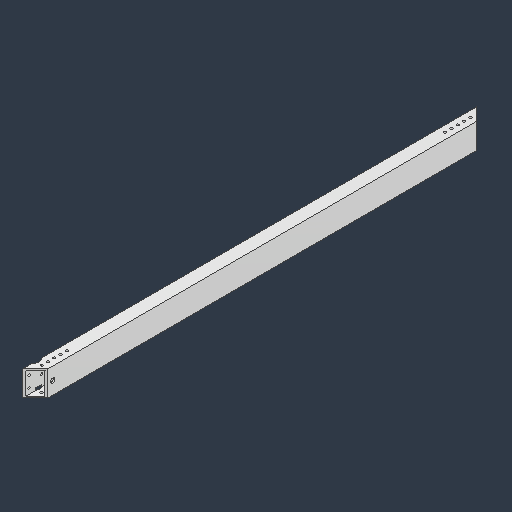
# Autodesk Inventor part: TUBE,ELEVATOR,SIDE,STAGE1
Saved by Autodesk Inventor 2024.3 (Build 283343000, 343)
## iProperties
Created: 2025-01-27
Part Number: TUBE,ELEVATOR,SIDE,STAGE1
Material: Aluminum 6061 T6 0 Cold Formed
Document SubType Name: Modeling
Designer: Jthib
Density: 2.7 g/cm^3
Appearance: Satin
Mass: 1058.01 g
Surface Area: 2496.4 cm^2
Volume: 391.854 cm^3
Mfg Approved By: John.Thibert
ILogicPurgeVersion: 0.0.0.0
OnSaveVersion: 3.4.3.0
OnSaveAssembly: COREAutomationManager
ModelCat: Uncategorized
MaterialName: Aluminum 6061 T6 0 Cold Formed
CN_MASS: 1.06
Author: Jthib
Autodesk Inventor part; units mm, degrees
ref_plane "YZ Plane" through (0, 0, 0) normal (1, 0, 0) x (0, 1, 0)
ref_plane "XZ Plane" through (0, 0, 0) normal (0, 1, 0) x (-1, 0, 0)
ref_plane "XY Plane" through (0, 0, 0) normal (0, 0, 1) x (1, 0, 0)
sketch "Sketch1" plane through (0, 0, 0) normal (0, 0, 1) x (1, 0, 0)
  line L0 (-12.7, -25.4) -> (12.7, -25.4)
  line L1 (12.7, -25.4) -> (12.7, 25.4)
  line L2 (12.7, 25.4) -> (-12.7, 25.4)
  line L3 (-12.7, 25.4) -> (-12.7, -25.4)
  line L4 (-12.7, -25.4) -> (12.7, 25.4) construction
  line L5 (12.7, -25.4) -> (-12.7, 25.4) construction
  line L6 (-9.525, 22.225) -> (9.525, 22.225)
  line L7 (9.525, 22.225) -> (9.525, -22.225)
  line L8 (9.525, -22.225) -> (-9.525, -22.225)
  line L9 (-9.525, -22.225) -> (-9.525, 22.225)
  point P0 (0, 0)
  dimension "d0" = 25.4
  dimension "d1" = 50.8
  dimension "d2" = 3.175
  constraints: 20 end point, 4 parallel, 2 midpoint, 2 perpendicular, 1 horizontal, 3 other
  measures "d0" distance of L2.end L1.end
  measures "d1" distance of L1.end L0.end
  measures "d2" distance between parallel lines of L2 L6
extrude "Extrusion1" add sketch "Sketch1" along normal mid plane 914.4
sketch "Sketch2" plane through (-12.7, -25.4, 457.2) normal (0, -1, 0) x (1, 0, 0)
  line L0 (25.4, 0) -> (25.4, -914.4) projected
  line L1 (0, 0) -> (25.4, 0) construction
  line L2 (0, -914.4) -> (0, 0) construction
  line L3 (25.4, -914.4) -> (0, -914.4) projected
  line L4 (0, -914.4) -> (25.4, -889)
  point P0 (12.7, -457.2)
  dimension "d6" = 45
  constraints: 2 end point, 1 point on line
  measures "d6" angle of L2 L4
extrude "Extrusion2" cut sketch "Sketch2" against normal through all
sketch "Sketch4" plane through (-12.7, -25.4, 457.2) normal (0, -1, 0) x (1, 0, 0)
  line L0 (0, -914.4) -> (0, 0) construction
  point P0 (12.7, -457.2)
  point P1 (12.7, -889)
  point P2 (12.7, -876.3)
  point P3 (12.7, -863.6)
  point P4 (12.7, -850.9)
  point P5 (12.7, -838.2)
  dimension "d9" = 12.7
  dimension "d10" = 25.4
  dimension "d13" = 12.7
  constraints: 1 vertical, 4 other
  measures "d9" distance from line of L0 point (12.7, -889)
  measures "d10" vertical distance of L0.start point (12.7, -889)
  measures "d13" distance of point (12.7, -889) point (12.7, -876.3)
hole "Hole1" at (0, -25.4, -431.8) at (0, -25.4, -419.1) at (0, -25.4, -406.4) at (0, -25.4, -393.7) at (0, -25.4, -381) direction (0, 1, 0) diameter 5.1054 end through all clearance for "Flat Head Machine Screw (82)" size "#10" standard "Ansi Unified Screw Threads"
mirror "Mirror1" about plane through (0, 0, 0) normal (0, 0, 1) of "Hole1", "Extrusion2"
sketch "Sketch5" plane through (12.7, -25.4, -431.8) normal (1, 0, 0) x (0, 0, -1)
  line L0 (-431.8, 25.4) -> (-854.075, 25.4) construction
  dimension "d25" = 422.275
  constraints: 2 end point, 1 coincident, 1 horizontal
  measures "d25" distance of L0.start L0.end
hole "Hole2" at (12.7, 0, 422.275) direction (-1, 0, 0) diameter 4.9784 end through all counterbore diameter 9.525 counterbore depth 12.7 clearance for "Socket Head Cap Screw" size "#10" standard "Ansi Unified Screw Threads"
sketch "Sketch6" plane through (-9.525, -22.225, -454.025) normal (1, 0, 0) x (0, 0, -1)
  circle A0 centre (-876.3, 22.225) radius 2.4892 construction
  line L0 (-876.3, 22.225) -> (-901.7, 22.225) construction
  line L1 (-901.7, 33.3375) -> (-901.7, 11.1125) construction
  point P0 (-454.025, 22.225)
  dimension "d33" = 25.4
  dimension "d34" = 22.225
  constraints: 4 end point, 1 horizontal, 1 midpoint, 1 vertical
  measures "d33" distance of L0.start L0.end
  measures "d34" distance of L1.start L1.end
hole "Hole3" at (-9.525, -11.1125, 447.675) at (-9.525, 11.1125, 447.675) direction (-1, 0, 0) diameter 4.9784 end through all clearance for "Socket Head Cap Screw" size "#10" standard "Ansi Unified Screw Threads"
sketch "Sketch7" plane through (-12.7, -25.4, -457.2) normal (0, -1, 0) x (1, 0, 0)
  circle A0 centre (-4.7625, 885.825) radius 9.525
  line L0 (0, 0) -> (0, 914.4) construction
  point P0 (12.7, 457.2)
  dimension "d42" = 4.7625
  dimension "d43" = 28.575
  dimension "d44" = 19.05
  constraints: 1 centre point
  measures "d42" distance from line of L0 A0.centre
  measures "d43" vertical distance of L0.end A0.centre
  measures "d44" diameter of A0
extrude "Extrusion3" cut sketch "Sketch7" against normal blind 7.62
mirror "Mirror2" about plane through (0, 0, 0) normal (0, 1, 0) of "Extrusion3"
body "Solid1"
